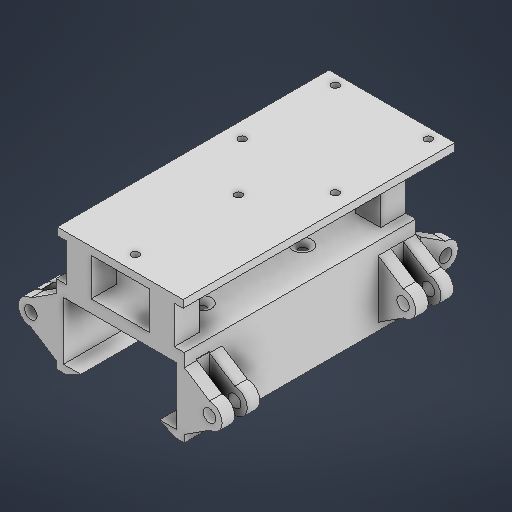
# Autodesk Inventor part: holder baterie+microcontroller+controller
Saved by Autodesk Inventor 2026.2 (Build 302298000, 298)
## iProperties
Created: 2026-03-28
Part Number: holder baterie+microcontroller+controller
Material: Generic
Document SubType Name: Modeling
Designer: Iosif
Density: 1 g/cm^3
Appearance: Default
Author: Iosif
## iProperties of the stored document holder baterie+microcontroller+controller_3DPrint.ipt
Created: 2026-03-28
Part Number: holder baterie+microcontroller+controller_3DPrint
Material: Generic
Document SubType Name: Modeling
Designer: Iosif
Density: 1 g/cm^3
Appearance: Default
Author: Iosif
Autodesk Inventor part; units mm, degrees
ref_plane "YZ Plane" through (0, 0, 0) normal (1, 0, 0) x (0, 1, 0)
ref_plane "XZ Plane" through (0, 0, 0) normal (0, 1, 0) x (-1, 0, 0)
ref_plane "XY Plane" through (0, 0, 0) normal (0, 0, 1) x (1, 0, 0)
sketch "Sketch1" plane through (0, 0, 0) normal (0, 1, 0) x (-1, 0, 0)
  line L0 (0, 0) -> (-43, 0)
  line L1 (-43, 0) -> (-43, -92)
  line L2 (-43, -92) -> (0, -92)
  line L3 (0, -92) -> (0, 0)
  line L4 (-43, -20.5) -> (0, -20.5) construction
  line L5 (-33.5, -92) -> (-33.5, 0) construction
  circle A0 centre (-33.5, -20.5) radius 1.75
  circle A1 centre (-33.5, -60.5) radius 1.75
  line L6 (-21.5, 0) -> (-21.5, -92) construction
  circle A2 centre (-9.5, -20.5) radius 1.75
  circle A3 centre (-9.5, -60.5) radius 1.75
  point P0 (-21.5, 0)
  dimension "d0" = 43
  dimension "d1" = 92
  dimension "d3" = 20.5
  dimension "d4" = 9.5
  dimension "d5" = 3.5
  dimension "d6" = 3.5
  dimension "d7" = 40
  dimension "d8" = 21.5
  constraints: 14 end point, 7 point on line, 4 centre point, 4 perpendicular, 3 midpoint, 2 parallel, 2 symmetric about line, 1 horizontal, 2 other
  measures "d0" distance of L2.end L1.end
  measures "d1" distance of L1.end L0.end
  measures "d3" distance from line of point (-21.5, 0) L4
  measures "d4" distance between parallel lines of L5 L1
  measures "d5" diameter of A0
  measures "d6" diameter of A1
  measures "d7" distance of A1.centre A0.centre
  measures "d8" distance between parallel lines of L1 L6
extrude "Extrusion1" add sketch "Sketch1" against normal blind 5
fillet "Fillet1" radius 2 1 edges at (11.25, 0, -20.5)
fillet "Fillet2" radius 2 1 edges at (35.25, 0, -20.5)
fillet "Fillet3" radius 2 1 edges at (11.25, 0, -60.5)
fillet "Fillet4" radius 2 1 edges at (35.25, 0, -60.5)
sketch "Sketch4" plane through (0, 0, 0) normal (0, 1, 0) x (1, 0, 0)
  line L0 (43, 0) -> (33, 0)
  line L1 (33, 0) -> (33, 10)
  line L2 (33, 10) -> (43, 10)
  line L3 (43, 10) -> (43, 0)
  line L4 (0, 0) -> (10, 0)
  line L5 (10, 0) -> (10, 10)
  line L6 (10, 10) -> (0, 10)
  line L7 (0, 10) -> (0, 0)
  circle A0 centre (33.5, 20.5) radius 1.75 projected
  line L8 (0, 92) -> (0, 0) construction
  line L9 (43, 0) -> (43, 92) construction
  circle A1 centre (33.5, 60.5) radius 1.75 construction
  line L10 (33.5, 60.5) -> (33.5, 71) construction
  line L11 (43, 92) -> (33, 92)
  line L12 (33, 92) -> (33, 82)
  line L13 (33, 82) -> (43, 82)
  line L14 (43, 82) -> (43, 92)
  line L15 (0, 92) -> (43, 92) projected
  line L16 (0, 92) -> (10, 92)
  line L17 (10, 92) -> (10, 82)
  line L18 (10, 82) -> (0, 82)
  line L19 (0, 82) -> (0, 92)
  point P0 (43, 71)
  point P1 (0, 71)
  dimension "d41" = 10
  dimension "d42" = 10
  dimension "d43" = 10
  dimension "d44" = 10
  dimension "d45" = 10.5
  dimension "d46" = 43
  dimension "d47" = 10.5
  dimension "d63" = 10
  dimension "d64" = 10
  dimension "d65" = 10
  dimension "d66" = 10
  constraints: 34 end point, 8 parallel, 4 horizontal, 4 perpendicular, 2 point on line, 1 vertical
  measures "d41" distance of L1.end L2.end
  measures "d42" distance of L0.end L1.end
  measures "d43" distance of L6.end L5.end
  measures "d44" distance of L5.end L4.end
  measures "d45" vertical distance of A0.centre L1.end
  measures "d46" distance between parallel lines of L8 L9
  measures "d47" distance of L10.start L10.end
  measures "d63" distance of L12.end L13.end
  measures "d64" distance of L12.end L11.end
  measures "d65" distance of L17.end L18.end
  measures "d66" distance of L16.end L17.end
extrude "Extrusion4" add sketch "Sketch4" along normal blind 15 contours L0 L1 L2 L3 | L7 L6 L5 L4
sketch "Sketch5" plane through (0, 15, 0) normal (0, 1, 0) x (1, 0, 0)
  line L0 (21.492, 108) -> (-3.508, 108)
  line L1 (-3.508, 108) -> (-3.508, 0)
  line L2 (-3.508, 0) -> (46.492, 0)
  line L3 (46.492, 0) -> (46.492, 108)
  line L4 (46.492, 108) -> (21.492, 108)
  line L5 (173.1726, 108) -> (43.7839, 108)
  line L6 (21.492, 108) -> (21.492, 16.1126)
  line L7 (-3.508, 104) -> (46.492, 104)
  line L8 (2.992, 108) -> (2.992, 0)
  line L9 (39.992, 108) -> (39.992, 0)
  circle A0 centre (2.992, 104) radius 1.5
  circle A1 centre (2.992, 67) radius 1.5
  circle A2 centre (39.992, 67) radius 1.5
  circle A3 centre (39.992, 104) radius 1.5
  line L10 (2.992, 0) -> (2.992, 33.1363)
  circle A4 centre (21.492, 6) radius 1.5
  circle A5 centre (21.492, 47) radius 1.5
  line L11 (43, 0) -> (43, 10) construction
  line L12 (0, 92) -> (0, 10) construction
  line L13 (43, 92) -> (0, 92) construction
  line L14 (62.9466, 54) -> (46.492, 54) construction
  circle A6 centre (21.492, 54) radius 3.5774 construction
  point P0 (0, 0)
  point P1 (0, 71)
  point P2 (-3.508, 0)
  dimension "d60" = 108
  dimension "d62" = 54
  constraints: 24 end point, 7 centre point, 1 point on line
  measures "d60" distance of L1.start L1.end
  measures "d62" distance between parallel lines of L0 L14
sketch "Sketch6" plane through (0, 0, 0) normal (0, 1, 0) x (1, 0, 0)
  line L0 (0, 92) -> (43, 92) projected
  line L1 (0, 92) -> (10, 92)
  line L2 (10, 92) -> (10, 82)
  line L3 (10, 82) -> (0, 82)
  line L4 (0, 82) -> (0, 92)
  line L5 (43, 92) -> (33, 92)
  line L6 (33, 92) -> (33, 82)
  line L7 (33, 82) -> (43, 82)
  line L8 (43, 82) -> (43, 92)
  point P0 (0, 0)
  dimension "d67" = 10
  dimension "d68" = 10
  dimension "d69" = 10
  dimension "d70" = 10
  constraints: 16 end point, 4 parallel, 2 horizontal, 2 perpendicular
  measures "d67" distance of L2.end L3.end
  measures "d68" distance of L1.end L2.end
  measures "d69" distance of L7.end L6.end
  measures "d70" distance of L6.end L5.end
extrude "Extrusion5" add sketch "Sketch6" along normal blind 15
extrude "Extrusion6" add sketch "Sketch5" along normal blind 3 contours L6 L7 A0 L8 L0 | L4 L9 A3 L7 L6 | L8 A0 L7 L1 L0 | L4 L3 L7 A3 L9 | L7 A3 L9 A2 L2 L8 A1 A0 | L7 A0 L8 A1 L2 L1 | L7 L3 L2 L9 A2 A3
sketch "Sketch8" plane through (0, -5, 0) normal (0, 0, 1) x (1, 0, 0)
  line L0 (0, 5) -> (-4, 5)
  line L1 (-4, 5) -> (-4, -0.0331)
  line L2 (-4, -0.0331) -> (-4, -23.0331)
  line L3 (-4, -23.0331) -> (-4, -26.0331)
  line L4 (-4, -26.0331) -> (0, -26.0331)
  line L5 (0, -26.0331) -> (5.8803, -23.0331)
  line L6 (5.8803, -23.0331) -> (0, -23.0331)
  line L7 (0, -23.0331) -> (-1.0369, -23.0331)
  line L8 (-1.0369, -23.0331) -> (-1.0369, -0.0331)
  line L9 (-1.0369, -0.0331) -> (0, -0.0331)
  line L10 (0, -0.0331) -> (0, 5)
  line L11 (43, 0) -> (0, 0) construction
  line L12 (21.5, 0) -> (21.5, -18.1993) construction
  line L13 (43, 5) -> (47, 5)
  line L14 (47, 5) -> (47, -0.0331)
  line L15 (47, -0.0331) -> (47, -23.0331)
  line L16 (47, -23.0331) -> (47, -26.0331)
  line L17 (47, -26.0331) -> (43, -26.0331)
  line L18 (43, -26.0331) -> (37.1197, -23.0331)
  line L19 (37.1197, -23.0331) -> (43, -23.0331)
  line L20 (43, -23.0331) -> (44.0369, -23.0331)
  line L21 (44.0369, -23.0331) -> (44.0369, -0.0331)
  line L22 (44.0369, -0.0331) -> (43, -0.0331)
  line L23 (43, -0.0331) -> (43, 5)
  dimension "d88" = 4
  dimension "d89" = 23
  dimension "d90" = 3
  constraints: 46 end point, 11 symmetric about line, 6 point on line, 5 perpendicular, 1 horizontal, 1 midpoint, 1 parallel, 1 vertical
  measures "d88" distance of L0.start L0.end
  measures "d89" distance of L1.end L2.end
  measures "d90" distance of L2.end L3.end
extrude "Extrusion8" add sketch "Sketch8" against normal blind 92
sketch "Sketch9" plane through (-3.508, 15, 0) normal (0, 0, 1) x (1, 0, 0)
  line L0 (-20.492, 0.0571) -> (-20.492, -49.9429) construction
  line L1 (-0.492, -15) -> (-0.492, -46.0331) construction
  line L2 (-20.492, -20.1715) -> (-20.492, -43.1715) construction
  line L3 (-0.492, -43.1715) -> (-0.492, -20.1715)
  line L4 (-20.492, -31.6715) -> (-7.992, -31.6715) construction
  circle A0 centre (-10.492, -31.6715) radius 2.5 construction
  circle A1 centre (-10.492, -31.6715) radius 2.5
  arc A2 (-10.492, -26.6715) -> (-10.492, -36.6715) centre (-10.492, -31.6715) ccw construction
  arc A3 (-10.492, -26.6715) -> (-10.492, -36.6715) centre (-10.492, -31.6715) ccw
  line L5 (-10.492, -26.6715) -> (-0.492, -20.1715)
  line L6 (-10.492, -36.6715) -> (-0.492, -43.1715)
  line L7 (3.508, -20) -> (46.508, -20) construction
  line L8 (25.008, -20) -> (25.008, -50) construction
  line L9 (25.008, -20) -> (55.008, -20) construction
  line L10 (50.508, -15) -> (50.508, -46.0331) construction
  line L11 (70.508, -20.1715) -> (70.508, -43.1715) construction
  line L12 (50.508, -43.1715) -> (50.508, -20.1715)
  line L13 (70.508, -31.6715) -> (50.508, -31.6715) construction
  circle A4 centre (60.508, -31.6715) radius 2.5 construction
  circle A5 centre (60.508, -31.6715) radius 2.5
  arc A6 (60.508, -36.6715) -> (60.508, -26.6715) centre (60.508, -31.6715) ccw construction
  arc A7 (60.508, -36.6715) -> (60.508, -26.6715) centre (60.508, -31.6715) ccw
  line L14 (60.508, -26.6715) -> (50.508, -20.1715)
  line L15 (60.508, -36.6715) -> (50.508, -43.1715)
  point P0 (3.508, -15)
  point P1 (-10.492, -43.1715)
  point P2 (-10.492, -20.1715)
  point P3 (-0.492, -31.6715)
  point P4 (60.508, -43.1715)
  point P5 (60.508, -20.1715)
  dimension "d93" = 50
  dimension "d94" = 20
  dimension "d95" = 23
  dimension "d96" = 5
  dimension "d97" = 10
  dimension "d98" = 30
  dimension "d99" = 90
  constraints: 28 end point, 16 symmetric about line, 8 point on circle, 7 centre point, 6 coincident, 4 point on line, 3 midpoint, 2 vertical, 1 concentric, 1 horizontal, 1 horizontal alignment, 1 parallel, 1 perpendicular, 7 other
  measures "d93" distance of L0.start L0.end
  measures "d94" distance between parallel lines of L1 L0
  measures "d95" distance of point (-10.492, -43.171) point (-10.492, -20.171)
  measures "d96" diameter of A0
  measures "d97" diameter of A2
  measures "d98" distance of L8.start L8.end
  measures "d99" angle of L8 L9
extrude "Extrusion9" add sketch "Sketch9" against normal blind 5
sketch "Sketch10" plane through (33, 0, -92) normal (0, 0, -1) x (-1, 0, 0)
  line L0 (-13.9444, 0.0358) -> (-13.9444, -30.9973) construction
  line L1 (-33.9534, -5.1357) -> (-33.9534, -28.1357) construction
  line L2 (-13.9444, -28.1357) -> (-13.9444, -5.1729)
  line L3 (-33.9534, -16.6357) -> (-21.4534, -16.6357) construction
  circle A0 centre (-23.9534, -16.6357) radius 2.5 construction
  circle A1 centre (-23.9534, -16.6357) radius 2.5
  arc A2 (-23.8967, -11.636) -> (-23.9534, -21.6357) centre (-23.9534, -16.6357) ccw construction
  arc A3 (-23.8967, -11.636) -> (-23.9534, -21.6357) centre (-23.9534, -16.6357) ccw
  line L4 (-23.8967, -11.636) -> (-13.9444, -5.1729)
  line L5 (-23.9534, -21.6357) -> (-13.9444, -28.1357)
  line L6 (-9.9715, -4.9642) -> (33.0285, -4.9642) construction
  line L7 (11.5285, -4.9642) -> (11.5285, -34.9642) construction
  line L8 (11.5285, -4.9642) -> (41.5285, -4.9642) construction
  line L9 (46.9537, -11.636) -> (37.0014, -5.1729)
  line L10 (57.0104, -16.6357) -> (37.0014, -16.6543) construction
  circle A4 centre (47.0104, -16.6357) radius 2.5 construction
  circle A5 centre (47.0104, -16.6357) radius 2.5
  arc A6 (47.0104, -21.6357) -> (46.9537, -11.636) centre (47.0104, -16.6357) ccw construction
  arc A7 (47.0104, -21.6357) -> (46.9537, -11.636) centre (47.0104, -16.6357) ccw
  line L11 (37.0014, 0.0358) -> (37.0014, -30.9973) construction
  line L12 (37.0014, -28.1357) -> (37.0014, -5.1729)
  line L13 (57.0104, -5.1357) -> (57.0104, -28.1357) construction
  line L14 (47.0104, -21.6357) -> (37.0014, -28.1357)
  point P0 (33, 0)
  point P1 (-9.9534, 0.0358)
  point P2 (-33.9534, -34.9071)
  point P3 (-23.9534, -28.1357)
  point P4 (-23.9534, -5.1357)
  point P5 (-13.9444, -16.6543)
  point P6 (37.0014, -16.6543)
  point P7 (47.0104, -28.1357)
  point P8 (47.0104, -5.1357)
  dimension "d102" = 23
  dimension "d103" = 5
  dimension "d104" = 10
  dimension "d105" = 30
  dimension "d106" = 90
  constraints: 28 end point, 16 symmetric about line, 8 point on circle, 7 centre point, 6 coincident, 3 midpoint, 3 point on line, 1 concentric, 1 horizontal, 1 horizontal alignment, 1 parallel, 1 perpendicular, 1 vertical, 10 other
  measures "d102" distance of point (-23.953, -28.136) point (-23.953, -5.136)
  measures "d103" diameter of A0
  measures "d104" diameter of A2
  measures "d105" distance of L8.start L7.end
  measures "d106" angle of L7 L8
extrude "Extrusion10" add sketch "Sketch10" against normal blind 5
sketch "Sketch11" plane through (33, 0, -87) normal (0, 0, 1) x (1, 0, 0)
  line L0 (-37.0689, 0.0762) -> (-37.0689, -30.9569) construction
  line L1 (-57.0689, -89.4568) -> (-57.0689, 56.2662) construction
  line L2 (-37.0689, -28.0953) -> (-37.0689, -5.0953)
  line L3 (-57.0689, -16.5953) -> (-44.5689, -16.5953) construction
  circle A0 centre (-47.0689, -16.5953) radius 2.5 construction
  circle A1 centre (-47.0689, -16.5953) radius 2.5
  arc A2 (-47.0689, -11.5953) -> (-47.0689, -21.5953) centre (-47.0689, -16.5953) ccw construction
  arc A3 (-47.0689, -11.5953) -> (-47.0689, -21.5953) centre (-47.0689, -16.5953) ccw
  line L4 (-47.0689, -11.5953) -> (-37.0689, -5.0953)
  line L5 (-47.0689, -21.5953) -> (-37.0689, -28.0953)
  line L6 (-33.0689, -4.9238) -> (9.9311, -4.9238) construction
  line L7 (-11.5689, -4.9238) -> (-11.5689, -34.9238) construction
  line L8 (-11.5689, -4.9238) -> (18.4311, -4.9238) construction
  line L9 (23.9311, -11.5953) -> (13.9311, -5.0953)
  line L10 (33.9311, -16.5953) -> (13.9311, -16.5953) construction
  circle A4 centre (23.9311, -16.5953) radius 2.5 construction
  circle A5 centre (23.9311, -16.5953) radius 2.5
  arc A6 (23.9311, -21.5953) -> (23.9311, -11.5953) centre (23.9311, -16.5953) ccw construction
  arc A7 (23.9311, -21.5953) -> (23.9311, -11.5953) centre (23.9311, -16.5953) ccw
  line L11 (13.9311, 0.0762) -> (13.9311, -30.9569) construction
  line L12 (13.9311, -28.0953) -> (13.9311, -5.0953)
  line L13 (33.9311, -89.4568) -> (33.9311, 56.2662) construction
  line L14 (23.9311, -21.5953) -> (13.9311, -28.0953)
  point P0 (-33, 0)
  point P1 (-33.0689, 0.0762)
  point P2 (-99.6317, 49.1914)
  point P3 (-47.0689, -28.0953)
  point P4 (-47.0689, -5.0953)
  point P5 (-37.0689, -16.5953)
  point P6 (23.9311, -28.0953)
  point P7 (23.9311, -5.0953)
  dimension "d109" = 23
  dimension "d110" = 5
  dimension "d111" = 10
  dimension "d112" = 30
  dimension "d113" = 90
  constraints: 30 end point, 16 symmetric about line, 8 point on circle, 7 centre point, 6 coincident, 3 midpoint, 3 point on line, 1 concentric, 1 horizontal, 1 horizontal alignment, 1 parallel, 1 perpendicular, 1 vertical, 7 other
  measures "d109" distance of point (-47.069, -28.095) point (-47.069, -5.095)
  measures "d110" diameter of A0
  measures "d111" diameter of A2
  measures "d112" distance of L7.start L7.end
  measures "d113" angle of L7 L8
sketch "Sketch12" plane through (33, 0, -87) normal (0, 0, 1) x (1, 0, 0)
  line L0 (-36.9987, 1.005) -> (-36.9987, -30.0281) construction
  line L1 (-11.4987, -4.995) -> (-11.4987, -34.995) construction
  line L2 (-32.9987, -4.995) -> (10.0013, -4.995) construction
  line L3 (-11.4987, -4.995) -> (18.5013, -4.995) construction
  line L4 (14.0013, 1.005) -> (14.0013, -30.0281) construction
  line L5 (-36.9987, -28.1665) -> (-36.9987, -4.1665)
  line L6 (-47.1415, -22.1563) -> (-36.9987, -28.1665)
  circle A0 centre (-47.0104, -16.6579) radius 2.5 construction
  circle A1 centre (-47.0104, -16.6579) radius 2.5
  arc A2 (-47.855, -11.2231) -> (-47.1415, -22.1563) centre (-47.0104, -16.6579) ccw
  arc A3 (-47.855, -11.2231) -> (-47.1415, -22.1563) centre (-47.0104, -16.6579) ccw construction
  line L7 (-56.9987, -16.1665) -> (-44.5134, -16.7807) construction
  line L8 (-47.855, -11.2231) -> (-36.9987, -4.1665)
  line L9 (24.8577, -11.2231) -> (14.0013, -4.1665)
  line L10 (14.0013, -28.1665) -> (14.0013, -4.1665)
  line L11 (24.1442, -22.1563) -> (14.0013, -28.1665)
  circle A4 centre (24.013, -16.6579) radius 2.5 construction
  circle A5 centre (24.013, -16.6579) radius 2.5
  arc A6 (24.1442, -22.1563) -> (24.8577, -11.2231) centre (24.013, -16.6579) ccw
  line L12 (34.0013, -16.1665) -> (14.0013, -16.1665) construction
  arc A7 (24.1442, -22.1563) -> (24.8577, -11.2231) centre (24.013, -16.6579) ccw construction
  point P0 (-33, 0)
  point P1 (-38.6377, -19.4638)
  point P2 (-38.7066, -19.3876)
  point P3 (-36.9987, -16.1665)
  point P4 (-46.9987, -28.1665)
  point P5 (-46.9987, -5.1665)
  point P6 (14.0013, -16.1665)
  point P7 (24.0013, -28.1665)
  point P8 (24.0013, -5.1665)
  dimension "d106" = 90
  dimension "d114" = 23
  dimension "d115" = 5
  dimension "d116" = 11
  dimension "d117" = 30
  dimension "d118" = 90
  constraints: 24 end point, 14 symmetric about line, 8 point on circle, 7 centre point, 6 coincident, 3 point on line, 2 midpoint, 1 concentric, 1 horizontal, 1 perpendicular, 1 vertical, 11 other
  measures "d114" distance of point (-46.999, -28.166) point (-46.999, -5.166)
  measures "d115" diameter of A0
  measures "d116" diameter of A3
  measures "d117" distance of L1.start L1.end
  measures "d118" angle of L1 L3
extrude "Extrusion11" add sketch "Sketch11" along normal blind 10
extrude "Extrusion12" cut sketch "Sketch12" along normal blind 5 contours L6 A2 L8 L5 | A1 | A6 L11 L10 L9 | A5
sketch "Sketch13" plane through (-3.508, 15, -5) normal (0, 0, -1) x (-1, 0, 0)
  line L0 (-50.4944, -14.9332) -> (-50.4944, -45.9663) construction
  line L1 (-24.9944, -19.9332) -> (-24.9944, -49.9332) construction
  line L2 (-46.4944, -19.9332) -> (-3.4944, -19.9332) construction
  line L3 (-24.9944, -19.9332) -> (5.0056, -19.9332) construction
  line L4 (0.5056, -14.9332) -> (0.5056, -45.9663) construction
  line L5 (-50.4944, -43.1047) -> (-50.4944, -20.1047)
  line L6 (-60.4944, -36.6047) -> (-50.4944, -43.1047)
  circle A0 centre (-60.4944, -31.6047) radius 2.5 construction
  circle A1 centre (-60.4944, -31.6047) radius 2.5
  arc A2 (-60.4944, -26.6047) -> (-60.4944, -36.6047) centre (-60.4944, -31.6047) ccw
  arc A3 (-60.4944, -26.6047) -> (-60.4944, -36.6047) centre (-60.4944, -31.6047) ccw construction
  line L7 (-70.4944, -31.6047) -> (-57.9944, -31.6047) construction
  line L8 (-60.4944, -26.6047) -> (-50.4944, -20.1047)
  line L9 (10.5056, -26.6047) -> (0.5056, -20.1047)
  line L10 (0.5056, -43.1047) -> (0.5056, -20.1047)
  line L11 (10.5056, -36.6047) -> (0.5056, -43.1047)
  circle A4 centre (10.5056, -31.6047) radius 2.5 construction
  circle A5 centre (10.5056, -31.6047) radius 2.5
  arc A6 (10.5056, -36.6047) -> (10.5056, -26.6047) centre (10.5056, -31.6047) ccw
  line L12 (20.5056, -31.6047) -> (0.5056, -31.6047) construction
  arc A7 (10.5056, -36.6047) -> (10.5056, -26.6047) centre (10.5056, -31.6047) ccw construction
  point P0 (-3.508, -15)
  point P1 (-46.4254, -15.0094)
  point P2 (-46.4944, -14.9332)
  point P3 (-50.4944, -31.6047)
  point P4 (-60.4944, -43.1047)
  point P5 (-60.4944, -20.1047)
  point P6 (10.5056, -43.1047)
  point P7 (10.5056, -20.1047)
  dimension "d123" = 23
  dimension "d124" = 5
  dimension "d125" = 10
  dimension "d126" = 30
  dimension "d127" = 90
  constraints: 26 end point, 14 symmetric about line, 8 point on circle, 7 centre point, 6 coincident, 3 point on line, 2 midpoint, 1 concentric, 1 horizontal, 1 horizontal alignment, 1 perpendicular, 1 vertical, 7 other
  measures "d123" distance of point (-60.494, -43.105) point (-60.494, -20.105)
  measures "d124" diameter of A0
  measures "d125" diameter of A3
  measures "d126" distance of L3.start L1.end
  measures "d127" angle of L1 L3
sketch "Sketch14" plane through (-3.508, 15, -5) normal (0, 0, -1) x (-1, 0, 0)
  circle A0 centre (10.4783, -31.6827) radius 2.5 construction
  circle A1 centre (10.4783, -31.6827) radius 2.5
  line L0 (11.4897, -26.7861) -> (0.7224, -19.6333)
  line L1 (12.7263, -36.1489) -> (1.0263, -43.7322)
  line L2 (20.9452, -32.0316) -> (0.8743, -31.6827) construction
  line L3 (-24.8227, -19.9434) -> (5.1773, -19.9434) construction
  line L4 (-24.8227, -19.9434) -> (-24.8227, -49.9434) construction
  line L5 (-46.3227, -19.9434) -> (-3.3227, -19.9434) construction
  line L6 (-50.6716, -43.7322) -> (-50.3678, -19.6333)
  line L7 (-53.5946, -21.9733) -> (-50.3678, -19.6333)
  circle A2 centre (-60.1237, -31.6827) radius 2.5
  line L8 (-50.2779, -14.8236) -> (-50.8577, -45.8512) construction
  line L9 (-70.5906, -32.0316) -> (-57.6251, -31.5995) construction
  circle A3 centre (-60.1237, -31.6827) radius 2.5 construction
  line L10 (1.0263, -43.7322) -> (0.7224, -19.6333)
  line L11 (0.6325, -14.8236) -> (1.2123, -45.8512) construction
  arc A4 (-65.1209, -31.8493) -> (-62.3716, -36.1489) centre (-60.1237, -31.6827) ccw construction
  arc A5 (12.7263, -36.1489) -> (11.4897, -26.7861) centre (10.4783, -31.6827) ccw
  arc A6 (12.7263, -36.1489) -> (11.4897, -26.7861) centre (10.4783, -31.6827) ccw construction
  line L12 (-61.366, -37.5317) -> (-50.6716, -43.7322)
  line L13 (-53.5946, -21.9733) -> (-62.6286, -23.0003)
  line L14 (-62.6286, -23.0003) -> (-67.4609, -33.4151)
  line L15 (-67.4609, -33.4151) -> (-64.8709, -37.9301)
  line L16 (-64.8709, -37.9301) -> (-61.366, -37.5317)
  point P0 (-3.508, -15)
  point P1 (-3.5208, -15.0102)
  point P2 (0.8743, -31.6827)
  point P3 (10.8618, -20.1149)
  point P4 (10.8618, -43.1149)
  point P5 (-46.4382, -15.0196)
  point P6 (-46.5071, -14.9434)
  point P7 (-50.5197, -31.6827)
  point P8 (-60.5071, -20.1149)
  point P9 (-60.5071, -43.1149)
  dimension "d128" = 23
  dimension "d129" = 5
  dimension "d130" = 10
  dimension "d131" = 30
  dimension "d132" = 90
  constraints: 32 end point, 12 symmetric about line, 6 centre point, 6 point on circle, 5 coincident, 4 point on line, 2 midpoint, 1 horizontal, 1 perpendicular, 1 vertical, 10 other
  measures "d128" distance of point (-60.507, -43.115) point (-60.507, -20.115)
  measures "d129" diameter of A3
  measures "d130" diameter of A4
  measures "d131" distance of L4.start L4.end
  measures "d132" angle of L4 L3
extrude "Extrusion13" add sketch "Sketch13" along normal blind 10
extrude "Extrusion14" cut sketch "Sketch14" along normal blind 5 contours A1 | A5 L1 L10 L0 | L12 L16 L15 L14 L13 L7 L6 | A2
sketch "Sketch15" plane through (47, -31.0331, 0) normal (1, 0, 0) x (0, 0, -1)
  line L0 (66.3515, 26.1608) -> (96.3515, 26.1608) construction
  line L1 (66.3515, 26.1608) -> (66.3515, -3.8392) construction
  line L2 (44.8515, 26.1608) -> (87.8515, 26.1608) construction
  line L3 (91.8244, 31.1608) -> (91.8244, 0.1277) construction
  line L4 (91.8244, 2.9893) -> (91.8244, 25.9521)
  line L5 (101.7767, 19.489) -> (91.8244, 25.9521)
  line L6 (101.8334, 9.4893) -> (91.8244, 2.9893)
  circle A0 centre (101.8334, 14.4893) radius 2.5 construction
  circle A1 centre (101.8334, 14.4893) radius 2.5
  arc A2 (101.8334, 9.4893) -> (101.7767, 19.489) centre (101.8334, 14.4893) ccw construction
  arc A3 (101.8334, 9.4893) -> (101.7767, 19.489) centre (101.8334, 14.4893) ccw
  line L7 (111.8334, 14.4893) -> (91.8244, 14.4707) construction
  line L8 (111.8334, 25.9893) -> (111.8334, 2.9893) construction
  point P0 (0, 31.0331)
  point P1 (87.823, 31.125)
  point P2 (91.8244, 14.4707)
  point P3 (101.8334, 2.9893)
  point P4 (101.8334, 25.9893)
  dimension "d140" = 30
  dimension "d141" = 90
  constraints: 16 end point, 4 centre point, 4 point on circle, 3 coincident, 1 horizontal, 1 midpoint, 1 perpendicular, 1 point on line, 1 vertical, 3 other
  measures "d140" distance of L0.start L1.end
  measures "d141" angle of L1 L0
extrude "Extrusion15" add sketch "Sketch15" along normal blind 2 and the other way blind 3
sketch "Sketch16" plane through (-4, -31.0331, -92) normal (-1, 0, 0) x (0, 0, 1)
  line L0 (0.3819, 31.2206) -> (0.3819, 0.1875) construction
  line L1 (25.8548, 26.2206) -> (55.8548, 26.2206) construction
  line L2 (25.8548, 26.2206) -> (25.8548, -3.7794) construction
  line L3 (4.3548, 26.2206) -> (47.3548, 26.2206) construction
  line L4 (-19.6271, 26.0491) -> (-19.6271, 3.0491) construction
  line L5 (0.3819, 3.0491) -> (0.3819, 26.0119)
  line L6 (-19.6271, 14.5491) -> (-7.1271, 14.5491) construction
  circle A0 centre (-9.6271, 14.5491) radius 2.5 construction
  circle A1 centre (-9.6271, 14.5491) radius 2.5
  arc A2 (-9.5704, 19.5488) -> (-9.6271, 9.5491) centre (-9.6271, 14.5491) ccw construction
  arc A3 (-9.5704, 19.5488) -> (-9.6271, 9.5491) centre (-9.6271, 14.5491) ccw
  line L7 (-9.5704, 19.5488) -> (0.3819, 26.0119)
  line L8 (-9.6271, 9.5491) -> (0.3819, 3.0491)
  point P0 (92, 31.0331)
  point P1 (4.3729, 31.2206)
  point P2 (-19.6271, -3.7223)
  point P3 (0.3819, 14.5305)
  point P4 (-9.6271, 3.0491)
  point P5 (-9.6271, 26.0491)
  dimension "d146" = 23
  dimension "d147" = 5
  dimension "d148" = 10
  dimension "d149" = 30
  dimension "d150" = 90
  constraints: 18 end point, 4 point on circle, 3 centre point, 3 coincident, 3 midpoint, 2 point on line, 1 concentric, 1 horizontal, 1 horizontal alignment, 1 parallel, 1 perpendicular, 1 vertical, 3 other
  measures "d146" distance of point (-9.627, 3.049) point (-9.627, 26.049)
  measures "d147" diameter of A0
  measures "d148" diameter of A2
  measures "d149" distance of L1.start L2.end
  measures "d150" angle of L2 L1
extrude "Extrusion16" add sketch "Sketch16" along normal blind 2 and the other way blind 3
body "Solid1"
